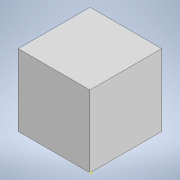
# Autodesk Inventor part: pawn
Saved by Autodesk Inventor 2021 (Build 250183000, 183)
## iProperties
Created: 2021-01-10
Part Number: pawn
Material: Generic
Document SubType Name: Modeling
Designer: Luke Kamols
Density: 1 g/cm^3
Appearance: Default
Author: Luke Kamols
Autodesk Inventor part; units mm, degrees
ref_plane "YZ Plane" through (0, 0, 0) normal (1, 0, 0) x (0, 1, 0)
ref_plane "XZ Plane" through (0, 0, 0) normal (0, 1, 0) x (-1, 0, 0)
ref_plane "XY Plane" through (0, 0, 0) normal (0, 0, 1) x (1, 0, 0)
sketch "Sketch1" plane through (0, 0, 0) normal (0, 1, 0) x (-1, 0, 0)
  point P0 (0, 0)
sketch "Sketch2" plane through (0, 0, 0) normal (0, 1, 0) x (-1, 0, 0)
  line L0 (0, 0) -> (16, 0)
  line L1 (16, 0) -> (16, -16)
  line L2 (16, -16) -> (0, -16)
  line L3 (0, -16) -> (0, 0)
  line L4 (0, 0) -> (0, -8)
  dimension "d1" = 16
  dimension "d2" = 16
  constraints: 10 end point, 2 parallel, 1 horizontal, 1 midpoint, 1 perpendicular
  measures "d1" distance of L1.end L2.end
  measures "d2" distance of L0.end L1.end
extrude "Extrusion1" add sketch "Sketch2" along normal blind 16
sketch "Sketch4" plane through (0, 0, 0) normal (0, -1, 0) x (1, 0, 0)
  line L0 (0, 0) -> (0, -16) projected
  line L1 (-16, -16) -> (-16, 0) projected
  line L2 (0, -16) -> (-16, -16) projected
  line L3 (0, 0) -> (0, -16) projected
  line L4 (-16, 0) -> (0, 0) projected
  line L5 (0, 0) -> (0, -16) projected
  line L6 (-16, -16) -> (-16, 0) projected
  line L7 (-8, -8) -> (-8, -11.3)
  line L8 (-8, -11.3) -> (-1.5, -11.3)
  line L9 (-1.5, -11.3) -> (-1.5, -4.7)
  line L10 (-1.5, -4.7) -> (-14.5, -4.7)
  line L11 (-14.5, -4.7) -> (-14.5, -11.3)
  line L12 (-14.5, -11.3) -> (-8, -11.3)
  line L13 (0, -8) -> (-8, -8)
  dimension "d28" = 3.3
  dimension "d29" = 6.5
  dimension "d30" = 6.6
  dimension "d31" = 13
  constraints: 14 end point, 5 perpendicular, 1 horizontal, 1 midpoint, 1 point on line, 1 vertical
  measures "d28" distance of L7.start L7.end
  measures "d29" distance of L7.end L8.end
  measures "d30" distance of L8.end L9.end
  measures "d31" distance of L9.end L10.end
extrude "Extrusion3" cut sketch "Sketch4" against normal blind 6.6 contours L13 L9 L8 L7 | L7 L12 L11 L10 L9 L13
chamfer "Chamfer1" distance 3.3 angle 45 2 edges at (-8, 6.6, -4.7) (-8, 6.6, -11.3)
body "Solid1"
